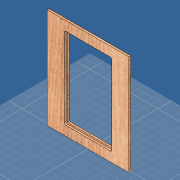
# Autodesk Inventor part: Flachfaltenfilter_Halter
Saved by Autodesk Inventor 2019 (Build 230136000, 136)
## iProperties
Created: 2020-08-02
Part Number: Flachfaltenfilter_Halter
Material: Generisch
Document SubType Name: Modeling
Designer: Stefan
Mass: 373.505 g
Surface Area: 1013.35 cm^2
Volume: 373.505 cm^3
Density: 1 g/cm^3
Appearance: Birke - natur - poliert
Author: Stefan
Autodesk Inventor part; units mm, degrees
ref_plane "YZ Plane" through (0, 0, 0) normal (1, 0, 0) x (0, 1, 0)
ref_plane "XZ Plane" through (0, 0, 0) normal (0, 1, 0) x (-1, 0, 0)
ref_plane "XY Plane" through (0, 0, 0) normal (0, 0, 1) x (1, 0, 0)
sketch "Skizze1" plane through (0, 0, 0) normal (0, 0, 1) x (1, 0, 0)
  line L0 (-65, 120) -> (65, 120)
  line L1 (70, 115) -> (70, -115)
  line L2 (65, -120) -> (-65, -120)
  line L3 (-70, -115) -> (-70, 115)
  line L4 (-70, 120) -> (70, -120) construction
  line L5 (70, 120) -> (-70, -120) construction
  arc A0 (-65, 120) -> (-70, 115) centre (-65, 115) ccw
  arc A1 (-70, -115) -> (-65, -120) centre (-65, -115) ccw
  arc A2 (65, -120) -> (70, -115) centre (65, -115) ccw
  arc A3 (70, 115) -> (65, 120) centre (65, 115) ccw
  line L6 (-64, -116) -> (64, -116)
  line L7 (66, -114) -> (66, 114)
  line L8 (64, 116) -> (-64, 116)
  line L9 (-66, 114) -> (-66, -114)
  line L10 (-66, -116) -> (66, 116) construction
  line L11 (66, -116) -> (-66, 116) construction
  arc A4 (66, 114) -> (64, 116) centre (64, 114) ccw
  arc A5 (64, -116) -> (66, -114) centre (64, -114) ccw
  arc A6 (-66, -114) -> (-64, -116) centre (-64, -114) ccw
  arc A7 (-64, 116) -> (-66, 114) centre (-64, 114) ccw
  line L12 (-62, 114) -> (62, 114)
  line L13 (64, 112) -> (64, -112)
  line L14 (62, -114) -> (-62, -114)
  line L15 (-64, -112) -> (-64, 112)
  line L16 (-64, 114) -> (64, -114) construction
  line L17 (64, 114) -> (-64, -114) construction
  arc A8 (64, 112) -> (62, 114) centre (62, 112) ccw
  arc A9 (62, -114) -> (64, -112) centre (62, -112) ccw
  arc A10 (-64, -112) -> (-62, -114) centre (-62, -112) ccw
  arc A11 (-62, 114) -> (-64, 112) centre (-62, 112) ccw
  line L18 (-120, -147.5) -> (120, -147.5)
  line L19 (120, -147.5) -> (120, 147.5)
  line L20 (120, 147.5) -> (-120, 147.5)
  line L21 (-120, 147.5) -> (-120, -147.5)
  line L22 (-120, -147.5) -> (120, 147.5) construction
  line L23 (120, -147.5) -> (-120, 147.5) construction
  line L24 (-105, -132.5) -> (105, -132.5)
  line L25 (105, -132.5) -> (105, 132.5)
  line L26 (105, 132.5) -> (-105, 132.5)
  line L27 (-105, 132.5) -> (-105, -132.5)
  line L28 (-105, -132.5) -> (105, 132.5) construction
  line L29 (105, -132.5) -> (-105, 132.5) construction
  point P0 (0, 0)
  point P1 (0, 0)
  point P2 (0, 0)
  dimension "d0" = 140
  dimension "d1" = 240
  dimension "d2" = 5
  dimension "d3" = 232
  dimension "d4" = 132
  dimension "d5" = 2
  dimension "d6" = 128
  dimension "d7" = 228
  dimension "d8" = 2
  dimension "d11" = 240
  dimension "d12" = 295
  dimension "d13" = 210
  dimension "d14" = 265
  constraints: 60 end point, 24 point on circle, 24 point on line, 24 tangent, 12 centre point, 11 midpoint, 10 parallel, 9 equal radius, 5 horizontal, 5 perpendicular, 1 coincident
  measures "d0" distance of L4.end L5.end
  measures "d1" distance of L5.start L4.end
  measures "d2" radius of A0
  measures "d3" distance of L11.start L10.end
  measures "d4" distance of L10.end L11.end
  measures "d5" radius of A4
  measures "d6" distance of L16.end L17.end
  measures "d7" distance of L17.start L16.end
  measures "d8" radius of A8
  measures "d11" distance of L20.end L19.end
  measures "d12" distance of L19.end L18.end
  measures "d13" distance of L26.end L25.end
  measures "d14" distance of L26.end L24.start
extrude "Extrusion1" add sketch "Skizze1" along normal blind 6 contours L21 L20 L19 L18 | L27 L26 L25 L24
extrude "Extrusion2" add sketch "Skizze1" against normal blind 6 contours L0 A3 L1 A2 L2 A1 L3 A0 | L27 L26 L25 L24
equation "\"d15\" = mdf_thickness"
equation "\"d17\" = mdf_thickness"
equation "\"kg_thickness\" = 4.9"
equation "\"ht_thickness\" = 1.9"
equation "\"case_thickness\" = 18"
equation "\"inner_thickness\" = 15"
equation "\"gap_fit\" = 0.1"
equation "\"gap_slide\" = 0.2"
equation "\"gap_air\" = 1"
equation "\"bore_diameter\" = 73"
equation "\"mdf_thickness\" = 6"
equation "\"tape_width\" = 15"
equation "\"tape_thickness\" = 3"
equation "\"inner_depth\" = 255"
